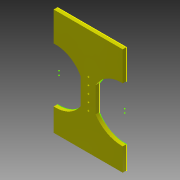
# Autodesk Inventor part: 知能ロボコン台座
Saved by Autodesk Inventor 2013 (Build 170138000, 138)
## iProperties
Created: 2014-05-31
Part Number: 知能ロボコン台座
Material: ABS プラスチック
Document SubType Name: Modeling
Designer: horumo136
Density: 1 g/cm^3
Author: horumo136
Autodesk Inventor part; units mm, degrees
note: some values were not read from the file. Chosen so that the rebuilt part matches the saved one: sketch regions of "押し出し3"; sketch regions of "押し出し4".
ref_plane "YZ Plane" through (0, 0, 0) normal (1, 0, 0) x (0, 1, 0)
ref_plane "XZ Plane" through (0, 0, 0) normal (0, 1, 0) x (-1, 0, 0)
ref_plane "XY Plane" through (0, 0, 0) normal (0, 0, 1) x (1, 0, 0)
sketch "スケッチ1" plane through (0, 0, 0) normal (0, 1, 0) x (-1, 0, 0)
  line L0 (0, 0) -> (0, 25)
  line L1 (0, 25) -> (0, 104.965)
  line L2 (0, 104.965) -> (0, 139.606)
  line L3 (-45, 25) -> (45, 25)
  line L4 (45, 25) -> (45, 0)
  line L5 (45, 0) -> (-45, 0)
  line L6 (-45, 0) -> (-45, 25)
  line L7 (-45, 25) -> (45, 0) construction
  line L8 (45, 25) -> (-45, 0) construction
  line L9 (-47, 28) -> (47, 28)
  line L10 (47, 28) -> (47, -3)
  line L11 (47, -3) -> (-47, -3)
  line L12 (-47, -3) -> (-47, 28)
  line L13 (-47, 28) -> (47, -3) construction
  line L14 (47, 28) -> (-47, -3) construction
  line L15 (-47, 142.2855) -> (47, 142.2855)
  line L16 (47, 142.2855) -> (47, 102.2855)
  line L17 (47, 102.2855) -> (-47, 102.2855)
  line L18 (-47, 102.2855) -> (-47, 142.2855)
  line L19 (-47, 142.2855) -> (47, 102.2855) construction
  line L20 (47, 142.2855) -> (-47, 102.2855) construction
  line L21 (-45, 139.606) -> (45, 139.606)
  line L22 (45, 139.606) -> (45, 104.965)
  line L23 (45, 104.965) -> (-45, 104.965)
  line L24 (-45, 104.965) -> (-45, 139.606)
  line L25 (-45, 139.606) -> (45, 104.965) construction
  line L26 (45, 139.606) -> (-45, 104.965) construction
  line L27 (-10, 28) -> (10, 28)
  line L28 (10, 28) -> (10, 102.2855)
  line L29 (10, 102.2855) -> (-10, 102.2855)
  line L30 (-10, 102.2855) -> (-10, 28)
  arc A0 (-10, 84.5837) -> (-47, 102.2855) centre (-46.0082, 56.8392) ccw
  arc A1 (-47, 28) -> (-10, 49.4601) centre (-44.5907, 66.4724) ccw
  arc A2 (47, 102.2855) -> (10, 84.5837) centre (46.0082, 56.8392) ccw
  arc A3 (10, 49.4601) -> (47, 28) centre (44.5907, 66.4724) ccw
  point P0 (0, 12.5)
  point P1 (0, 12.5)
  point P2 (0, 122.2855)
  point P3 (0, 122.2855)
  dimension "d0" = 25
  dimension "d1" = 79.965
  dimension "d2" = 34.641
  dimension "d3" = 90
  dimension "d4" = 94
  dimension "d5" = 31
  dimension "d6" = 94
  dimension "d7" = 40
  dimension "d8" = 90
  dimension "d9" = 20
  dimension "d10" = 10
  constraints: 62 end point, 13 midpoint, 10 parallel, 8 point on circle, 5 horizontal, 5 perpendicular, 4 centre point, 4 point on line, 4 symmetric about line, 2 collinear, 1 vertical, 2 other
  measures "d0" distance of L0.start L0.end
  measures "d1" distance of L0.end L1.end
  measures "d2" distance of L1.end L2.end
  measures "d3" distance of L4.end L5.end
  measures "d4" distance of L10.end L11.end
  measures "d5" distance of L9.end L10.end
  measures "d6" distance of L16.end L17.end
  measures "d7" distance of L15.end L16.end
  measures "d8" distance of L22.end L23.end
  measures "d9" distance between parallel lines of L28 L30
  measures "d10" distance between parallel lines of L1 L30
extrude "押し出し1" add sketch "スケッチ1" along normal blind 3 contours L9 L30 L17 L1 | L9 A3 L10 L11 L12 A1 | L1 L17 L28 L9 | L17 A0 L18 L15 L16 A2 | A1 L9 | L9 A3 | A2 L17 | L17 A0
sketch "スケッチ2" plane through (0, 3, 0) normal (0, 1, 0) x (1, 0, 0)
  line L0 (-45, -139.606) -> (-45, -104.965) projected
  line L1 (-45, -104.965) -> (45, -104.965) projected
  line L2 (45, -104.965) -> (45, -139.606) projected
  line L3 (45, -139.606) -> (-45, -139.606) projected
  line L4 (-45, -25) -> (-45, 0) projected
  line L5 (-45, 0) -> (45, 0) projected
  line L6 (45, 0) -> (45, -25) projected
  line L7 (45, -25) -> (-45, -25) projected
  line L8 (-10, -28) -> (-10, -102.2855) projected
  line L9 (-10, -102.2855) -> (-47, -102.2855) projected
  line L10 (-47, -102.2855) -> (-47, -142.2855) projected
  line L11 (-47, -142.2855) -> (47, -142.2855) projected
  line L12 (47, -142.2855) -> (47, -102.2855) projected
  line L13 (47, -102.2855) -> (10, -102.2855) projected
  line L14 (10, -102.2855) -> (10, -28) projected
  line L15 (10, -28) -> (47, -28) projected
  line L16 (47, -28) -> (47, 3) projected
  line L17 (47, 3) -> (-47, 3) projected
  line L18 (-47, 3) -> (-47, -28) projected
  line L19 (-47, -28) -> (-10, -28) projected
  arc A0 (-10, -47.2222) -> (-47, -28) centre (-44.6937, -68.7817) ccw
  arc A1 (-47, -102.2855) -> (-10, -81.2921) centre (-44.5262, -63.5433) ccw
  line L20 (0, -57.408) -> (0, -62.3253)
  arc A2 (47, -28) -> (10, -47.2222) centre (44.6937, -68.7817) ccw
  arc A3 (10, -81.2921) -> (47, -102.2855) centre (44.5262, -63.5433) ccw
  arc A4 (-10, -47.2222) -> (-47, -28) centre (-44.6937, -68.7817) ccw
  arc A5 (-47, -102.2855) -> (-10, -81.2921) centre (-44.5262, -63.5433) ccw
  arc A6 (47, -28) -> (10, -47.2222) centre (44.6937, -68.7817) ccw
  arc A7 (10, -81.2921) -> (47, -102.2855) centre (44.5262, -63.5433) ccw
  point P0 (0, 0)
  constraints: 16 point on circle, 8 centre point, 5 concentric, 4 symmetric about line, 2 end point, 2 point on line, 1 perpendicular, 2 other
sketch "スケッチ3" plane through (0, 3, 0) normal (0, 1, 0) x (1, 0, 0)
  line L0 (-45, -139.606) -> (-45, -104.965) projected
  line L1 (-45, -104.965) -> (45, -104.965) projected
  line L2 (45, -104.965) -> (45, -139.606) projected
  line L3 (45, -139.606) -> (-45, -139.606) projected
  line L4 (-45, -25) -> (-45, 0) projected
  line L5 (-45, 0) -> (45, 0) projected
  line L6 (45, 0) -> (45, -25) projected
  line L7 (45, -25) -> (-45, -25) projected
  line L8 (-10, -28) -> (-10, -102.2855) projected
  line L9 (-10, -102.2855) -> (-47, -102.2855) projected
  line L10 (-47, -102.2855) -> (-47, -142.2855) projected
  line L11 (-47, -142.2855) -> (47, -142.2855) projected
  line L12 (47, -142.2855) -> (47, -102.2855) projected
  line L13 (47, -102.2855) -> (10, -102.2855) projected
  line L14 (10, -102.2855) -> (10, -28) projected
  line L15 (10, -28) -> (47, -28) projected
  line L16 (47, -28) -> (47, 3) projected
  line L17 (47, 3) -> (-47, 3) projected
  line L18 (-47, 3) -> (-47, -28) projected
  line L19 (-47, -28) -> (-10, -28) projected
  arc A0 (-10, -47.2222) -> (-47, -28) centre (-44.6589, -68.7147) ccw
  arc A1 (47, -28) -> (10, -47.2222) centre (45.0843, -69.5335) ccw
  arc A2 (10, -81.5262) -> (47, -102.2855) centre (44.8559, -62.7542) ccw
  arc A3 (-47, -102.2855) -> (-10, -81.5262) centre (-44.3224, -63.705) ccw
  point P0 (0, 0)
  constraints: 8 point on circle, 4 centre point, 4 point on line
extrude "押し出し3" add sketch "スケッチ3" against normal blind 3 contours L19 A0 L18 L17 L16 A1 L15 L14 L13 A2 L12 L11 L10 A3 L9 L8 | L8 A0 L19 | L19 A0 | L8 L9 A3 | A3 L9 | L15 A1 | A2 L13
sketch "スケッチ4" plane through (0, 3, 0) normal (0, 1, 0) x (1, 0, 0)
  line L0 (-45, -139.606) -> (-45, -104.965) projected
  line L1 (-45, -104.965) -> (45, -104.965) projected
  line L2 (45, -104.965) -> (45, -139.606) projected
  line L3 (45, -139.606) -> (-45, -139.606) projected
  line L4 (-45, -25) -> (-45, 0) projected
  line L5 (-45, 0) -> (45, 0) projected
  line L6 (45, 0) -> (45, -25) projected
  line L7 (45, -25) -> (-45, -25) projected
  line L8 (-10, -47.2222) -> (-10, -81.5262) projected
  arc A0 (-41.6448, -102.2855) -> (-10, -81.5262) centre (-44.3224, -63.705) ccw projected
  line L9 (-41.6448, -102.2855) -> (-47, -102.2855) projected
  line L10 (-47, -102.2855) -> (-47, -142.2855) projected
  line L11 (-47, -142.2855) -> (47, -142.2855) projected
  line L12 (47, -142.2855) -> (47, -102.2855) projected
  line L13 (47, -102.2855) -> (10, -102.2855) projected
  line L14 (10, -102.2855) -> (10, -28) projected
  line L15 (10, -28) -> (47, -28) projected
  line L16 (47, -28) -> (47, 3) projected
  line L17 (47, 3) -> (-47, 3) projected
  line L18 (-47, 3) -> (-47, -28) projected
  line L19 (-47, -28) -> (-42.3178, -28) projected
  arc A1 (-10, -47.2222) -> (-42.3178, -28) centre (-44.6589, -68.7147) ccw projected
  arc A2 (47, -28) -> (10, -47.2222) centre (45.7708, -70.8549) ccw
  arc A3 (10, -81.5262) -> (47, -102.2855) centre (45.1409, -62.2461) ccw
  point P0 (0, 0)
  constraints: 4 point on circle, 2 centre point, 2 point on line
extrude "押し出し4" add sketch "スケッチ4" against normal blind 3
sketch "スケッチ5" plane through (0, 0, 0) normal (0, -1, 0) x (1, 0, 0)
  arc A0 (43.2819, 102.2855) -> (10, 81.5262) centre (45.1409, 62.2461) ccw projected
  line L0 (47, 102.2855) -> (43.2819, 102.2855) projected
  line L1 (47, 142.2855) -> (47, 102.2855) projected
  line L2 (-47, 142.2855) -> (47, 142.2855) projected
  line L3 (-47, 102.2855) -> (-47, 142.2855) projected
  line L4 (-41.6448, 102.2855) -> (-47, 102.2855) projected
  arc A1 (-10, 81.5262) -> (-41.6448, 102.2855) centre (-44.3224, 63.705) ccw projected
  line L5 (-10, 47.2222) -> (-10, 81.5262) projected
  arc A2 (-42.3178, 28) -> (-10, 47.2222) centre (-44.6589, 68.7147) ccw projected
  line L6 (-47, 28) -> (-42.3178, 28) projected
  line L7 (-47, -3) -> (-47, 28) projected
  line L8 (47, -3) -> (-47, -3) projected
  line L9 (47, 28) -> (47, -3) projected
  line L10 (44.5416, 28) -> (47, 28) projected
  arc A3 (10, 47.2222) -> (44.5416, 28) centre (45.7708, 70.8549) ccw projected
  line L11 (10, 81.5262) -> (10, 47.2222) projected
  point P0 (0, 0)
extrude "押し出し5" add sketch "スケッチ5" along normal blind 2
sketch "スケッチ6" plane through (0, 3, 0) normal (0, 1, 0) x (1, 0, 0)
  line L0 (45, -104.965) -> (-45, -104.965)
  line L1 (-45, -104.965) -> (-45, -104.865)
  line L2 (-45, -104.865) -> (45, -104.865)
  line L3 (45, -104.865) -> (45, -104.965)
  point P0 (0, 0)
  dimension "d21" = 0.1
  constraints: 8 end point, 2 parallel, 1 horizontal, 1 perpendicular
  measures "d21" distance of L0.end L1.end
extrude "押し出し6" cut sketch "スケッチ6" against normal blind 3
sketch "スケッチ7" plane through (-10, 3, 47.2222) normal (-1, 0, 0) x (0, 0, 1)
  line L0 (34.3041, -5) -> (0, -5) projected
  line L1 (57.6402, 0) -> (44.0812, 0)
  line L2 (44.0812, 0) -> (54.2504, 5.8712)
  line L3 (57.6402, 0) -> (54.2504, 5.8712)
  point P0 (-47.2222, -3)
  dimension "d24" = 30
  constraints: 6 end point, 1 parallel, 1 perpendicular
  measures "d24" angle of L1 L2
extrude "押し出し7" add sketch "スケッチ7" against normal blind 20
sketch "スケッチ8" plane through (-10, 3, 47.2222) normal (-1, 0, 0) x (0, 0, 1)
  line L0 (57.6402, 0) -> (44.0812, 0) projected
  line L1 (54.2504, 5.8712) -> (57.6402, 0) projected
  line L2 (44.0812, 0) -> (54.2504, 5.8712) projected
  line L3 (57.6402, 0) -> (48.1987, 16.3532)
  line L4 (44.0812, 13.9759) -> (44.0812, 0)
  line L5 (44.0812, 13.9759) -> (48.1987, 16.3532)
  point P0 (-47.2222, -3)
  dimension "d27" = 18.883
  constraints: 6 end point, 3 perpendicular
  measures "d27" distance of L0.start L3.end
extrude "押し出し8" add sketch "スケッチ8" against normal blind 20 contours L4 L5 L3 L2
sketch "スケッチ9" plane through (-10, 3, 47.2222) normal (-1, 0, 0) x (0, 0, 1)
  line L0 (48.1987, 16.3532) -> (44.0812, 13.9759) projected
  line L1 (44.0812, 13.9759) -> (44.0812, 0) projected
  line L2 (48.1987, 16.3532) -> (47.6747, 17.2608)
  line L3 (47.6747, 17.2608) -> (43.5572, 14.8835)
  line L4 (43.5572, 14.8835) -> (44.0812, 13.9759)
  line L5 (44.0812, 13.9759) -> (48.1987, 16.3532)
  line L6 (44.0812, 13.9759) -> (44.0812, 15.1861)
  point P0 (-47.2222, -3)
  dimension "d30" = 1.048
  constraints: 10 end point, 2 parallel, 2 perpendicular, 1 collinear, 1 point on line
  measures "d30" distance of L0.start L2.end
extrude "押し出し9" add sketch "スケッチ9" against normal blind 20 contours L0 L6 L3 L2
sketch "スケッチ10" plane through (-10, 3, 47.2222) normal (-1, 0, 0) x (0, 0, 1)
  line L0 (57.6402, 0) -> (44.0812, 0) projected
  line L1 (57.6402, 0) -> (47.6747, 17.2608) projected
  line L2 (47.6747, 17.2608) -> (44.0812, 15.1861) projected
  line L3 (44.0812, 15.1861) -> (44.0812, 0) projected
  point P0 (-47.2222, -3)
extrude "押し出し10" cut sketch "スケッチ10" against normal blind 20
sketch "スケッチ11" plane through (0, -2, 0) normal (0, -1, 0) x (1, 0, 0)
  line L0 (-47, -3) -> (47, -3) projected
  line L1 (10, 47.2222) -> (10, 81.5262) projected
  line L2 (0, -3) -> (0, 47)
  line L3 (0, 47) -> (0, 57)
  line L4 (0, 57) -> (0, 67)
  line L5 (0, 67) -> (0, 77)
  line L6 (0, 77) -> (0, 87)
  circle A0 centre (0, 47) radius 1.5
  circle A1 centre (0, 57) radius 1.5
  circle A2 centre (0, 67) radius 1.5
  circle A3 centre (0, 77) radius 1.5
  circle A4 centre (0, 87) radius 1.5
  point P0 (0, 0)
  dimension "d35" = 50
  dimension "d36" = 10
  dimension "d37" = 10
  dimension "d38" = 10
  dimension "d39" = 10
  dimension "d40" = 3
  dimension "d41" = 3
  dimension "d42" = 3
  dimension "d43" = 3
  dimension "d44" = 3
  constraints: 10 end point, 5 centre point, 5 coincident, 4 collinear, 1 midpoint, 1 parallel
  measures "d35" distance of L2.start L2.end
  measures "d36" distance of L2.end L3.end
  measures "d37" distance of L3.end L4.end
  measures "d38" distance of L4.end L5.end
  measures "d39" distance of L5.end L6.end
  measures "d40" diameter of A0
  measures "d41" diameter of A1
  measures "d42" diameter of A2
  measures "d43" diameter of A3
  measures "d44" diameter of A4
hole "穴1" at (0, -2, 87) at (0, -2, 77) at (0, -2, 67) at (0, -2, 57) at (0, -2, 47) direction (0, 1, 0) diameter 3 depth 8 tip angle 118
